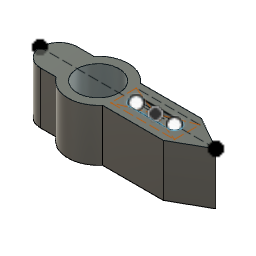
snafu-countdown-timer-arrow-v5 (Autodesk Fusion 360 design; units mm, degrees)
Autodesk Fusion 360 part; units mm, degrees
sketch "Sketch1" plane through (0, 0, 0) normal (0, 1, 0) x (1, 0, 0)
  line L0 (-20.3838, 3.2056) -> (-17.6853, 3.2056)
  line L1 (-20.3584, -2.5911) -> (-17.8516, -2.5911)
  line L2 (-10.3249, 3.1994) -> (-0.7249, 3.1994)
  line L3 (-0.7249, 3.1994) -> (4.589, 0.1994)
  line L4 (4.589, 0.1994) -> (-0.7249, -2.8006)
  line L5 (-0.7249, -2.8006) -> (-10.3249, -2.8006)
  arc A0 (-20.1646, 3.2056) -> (-20.19, -2.5911) centre (-20.2742, 0.3077) ccw
  arc A1 (-10.3249, 3.1994) -> (-17.6853, 3.2056) centre (-14.0077, 0.1994) ccw
  arc A2 (-17.8516, -2.5911) -> (-10.3249, -2.8006) centre (-14.0077, 0.1994) ccw
  line L6 (-22.911, 1.5149) -> (3.7873, -2.43) construction
  dimension "d1" = 5.8
  dimension "d2" = 9.5
  dimension "d4" = 27.5
  dimension "d32" = 6
  dimension "d33" = 9.6
  dimension "d34" = 9
  constraint coincident L0.start A0
  constraint horizontal L0
  constraint coincident L1.start A0
  constraint coincident L1.end A1
  constraint parallel L0 L1
  constraint coincident L6.start A0
  constraint parallel L0 L2
  constraint parallel L2 L5
  constraint concentric A1 A2
  constraint coincident L0 A0.start
  constraint coincident L1 A0.end
  constraint equal L3 L4
  constraint equal L2 L5
  constraint vertical L5.end L2.start
  constraint coincident A1.centre L6
  measures "d1" diameter of A0
  measures "d2" diameter of A1
  measures "d4" horizontal distance of L6.start L3.end
  measures "d32" distance of L2 L5
  measures "d33" distance of L2.end L2.start
  measures "d34" distance of A1.centre L6.start
extrude "Extrude1" add sketch "Sketch1" along normal blind 8.2
sketch "Sketch2" plane through (0, 8.2, 0) normal (0, 1, 0) x (-1, 0, 0)
  arc A0 (20.3838, -3.2056) -> (20.3584, 2.5911) centre (20.2742, -0.3077) ccw
  line L0 (20.3584, 2.5911) -> (17.8516, 2.5911)
  arc A1 (17.8516, 2.5911) -> (10.3249, 2.8006) centre (14.0077, -0.1994) ccw
  line L1 (10.3249, 2.8006) -> (0.7249, 2.8006)
  line L2 (0.7249, 2.8006) -> (-4.589, -0.1994)
  line L3 (-4.589, -0.1994) -> (0.7249, -3.1994)
  line L4 (0.7249, -3.1994) -> (10.3249, -3.1994)
  arc A2 (10.3249, -3.1994) -> (17.6853, -3.2056) centre (14.0077, -0.1994) ccw
  line L5 (17.6853, -3.2056) -> (20.3838, -3.2056)
  circle A3 centre (14.0077, -0.1994) radius 3.3
  dimension "d9" = 6.6
  constraint concentric A1 A3
  measures "d9" diameter of A3
extrude "Extrude2" cut sketch "Sketch2" against normal blind 5 contours A3
sketch "Sketch3" plane through (0, 3.2, 0) normal (0, 1, 0) x (-1, 0, 0)
  circle A0 centre (14.0077, -0.1994) radius 3.3
  line L0 (12.7077, -1.4994) -> (15.3077, -1.4994)
  line L1 (15.3077, -1.4994) -> (15.3077, 1.1006)
  line L2 (15.3077, 1.1006) -> (12.7077, 1.1006)
  line L3 (12.7077, 1.1006) -> (12.7077, -1.4994)
  line L4 (12.7077, -1.4994) -> (15.3077, 1.1006) construction
  line L5 (15.3077, -1.4994) -> (12.7077, 1.1006) construction
  point P0 (14.0077, -0.1994)
  dimension "d12" = 2.6
  constraint horizontal L0
  constraint perpendicular L0 L1
  constraint parallel L0 L2
  constraint parallel L1 L3
  constraint coincident L4 P0
  constraint coincident L5 P0
  constraint coincident P0 A0.centre
  constraint equal L1 L2
  measures "d12" distance of L0.end L1.end
extrude "Extrude3" cut sketch "Sketch3" against normal blind 13 contours L0 L1 L2 L3
sketch "Sketch6" plane through (0, 8.2, 0) normal (0, 1, 0) x (-1, 0, 0)
  circle A0 centre (14.0077, -0.1994) radius 3.3
  arc A1 (20.3838, -3.2056) -> (20.3584, 2.5911) centre (20.2742, -0.3077) ccw
  line L0 (20.3584, 2.5911) -> (17.8516, 2.5911)
  arc A2 (17.8516, 2.5911) -> (10.3249, 2.8006) centre (14.0077, -0.1994) ccw
  line L1 (10.3249, 2.8006) -> (0.7249, 2.8006)
  line L2 (0.7249, 2.8006) -> (-4.589, -0.1994)
  line L3 (-4.589, -0.1994) -> (0.7249, -3.1994)
  line L4 (0.7249, -3.1994) -> (10.3249, -3.1994)
  arc A3 (10.3249, -3.1994) -> (17.6853, -3.2056) centre (14.0077, -0.1994) ccw
  line L5 (17.6853, -3.2056) -> (20.3838, -3.2056)
  line L6 (-0.0396, -2.1994) -> (9.9928, -2.1994) construction
  line L7 (9.9928, -2.1994) -> (9.9928, 1.8006) construction
  line L8 (9.9928, 1.8006) -> (-0.0396, 1.8006) construction
  line L9 (-0.0396, 1.8006) -> (-0.0396, -2.1994) construction
  line L10 (-0.0396, -2.1994) -> (9.9928, 1.8006) construction
  line L11 (9.9928, -2.1994) -> (-0.0396, 1.8006) construction
  line L12 (7.9828, 0.8006) -> (1.9704, 0.8006)
  line L13 (0.9604, -0.2094) -> (0.9604, -0.1894)
  line L14 (1.9704, -1.1994) -> (7.9828, -1.1994)
  line L15 (8.9928, -0.1894) -> (8.9928, -0.2094)
  arc A4 (0.9604, -0.1894) -> (1.9704, -1.1994) centre (1.9704, -0.1894) ccw
  arc A5 (1.9704, 0.8006) -> (0.9604, -0.2094) centre (1.9704, -0.2094) ccw
  arc A6 (8.9928, -0.2094) -> (7.9828, 0.8006) centre (7.9828, -0.2094) ccw
  arc A7 (7.9828, -1.1994) -> (8.9928, -0.1894) centre (7.9828, -0.1894) ccw
  line L16 (-4.589, -0.1994) -> (8.9928, -0.1994) construction
  line L17 (9.9928, -0.1994) -> (23.1722, -0.1994) construction
  point P0 (4.9766, -0.1994)
  dimension "d28" = 1.01
  dimension "d29" = 2
  constraint coincident L2.end L3.start
  constraint coincident A1 L17.end
  constraint horizontal L16
  constraint horizontal L6
  constraint perpendicular L6 L7
  constraint parallel L6 L8
  constraint parallel L7 L9
  constraint coincident L10 P0
  constraint coincident L11 P0
  constraint coincident P0 L16
  constraint tangent L13 A4
  constraint tangent L14 A4
  constraint tangent L12 A5
  constraint tangent L13 A5
  constraint equal A4 A5
  constraint tangent L12 A6
  constraint tangent L15 A6
  constraint equal A4 A6
  constraint tangent L14 A7
  constraint tangent L15 A7
  constraint equal A4 A7
  constraint coincident L15 L16.end
  constraint coincident L7 L17.start
  constraint collinear L16 L17
  measures "d28" radius of A4
  measures "d29" distance of L4 L14
extrude "Extrude4" cut sketch "Sketch6" against normal blind 0.6 contours L12 L13 L14 L15 A4 A5 A6 A7
sketch "Sketch9" plane through (0, 0, 0) normal (0, -1, 0) x (1, 0, 0)
  line L0 (-12.7077, -1.4994) -> (-15.3077, -1.4994)
  line L1 (-15.3077, -1.4994) -> (-15.3077, 1.1006)
  line L2 (-15.3077, 1.1006) -> (-12.7077, 1.1006)
  line L3 (-12.7077, 1.1006) -> (-12.7077, -1.4994)
  arc A0 (-20.3584, 2.5911) -> (-20.3838, -3.2056) centre (-20.2742, -0.3077) ccw
  line L4 (-20.3838, -3.2056) -> (-17.6853, -3.2056)
  arc A1 (-17.6853, -3.2056) -> (-10.3249, -3.1994) centre (-14.0077, -0.1994) ccw
  line L5 (-10.3249, -3.1994) -> (-0.7249, -3.1994)
  line L6 (-0.7249, -3.1994) -> (4.589, -0.1994)
  line L7 (4.589, -0.1994) -> (-0.7249, 2.8006)
  line L8 (-0.7249, 2.8006) -> (-10.3249, 2.8006)
  arc A2 (-10.3249, 2.8006) -> (-17.8516, 2.5911) centre (-14.0077, -0.1994) ccw
  line L9 (-17.8516, 2.5911) -> (-20.3584, 2.5911)
  line L10 (-0.7249, -3.1994) -> (-10.3249, -3.1994)
  line L11 (-10.3249, 2.8006) -> (-0.7249, 2.8006)
  line L12 (-0.7249, 2.8006) -> (4.589, -0.1994)
  line L13 (4.589, -0.1994) -> (-0.7249, -3.1994)
  line L14 (-10.3249, -3.1994) -> (-10.3249, 2.8006) construction
  line L15 (-1.0403, -1.9994) -> (2.1481, -0.1994)
  line L16 (2.1481, -0.1994) -> (-1.0403, 1.6006)
  line L17 (-1.0403, 1.6006) -> (-9.1249, 1.6006)
  line L18 (-9.1249, -1.9994) -> (-9.1249, 1.6006)
  line L19 (-9.1249, -1.9994) -> (-1.0403, -1.9994)
  point P0 (-10.3249, -3.1994)
  point P1 (-0.7249, -3.1994)
  point P2 (4.589, -0.1994)
  point P3 (-0.7249, 2.8006)
  point P4 (-10.3249, 2.8006)
  dimension "d35" = -1.2
  constraint coincident P0 A1.end
  constraint coincident P4 L8.end
extrude "Extrude5" cut sketch "Sketch9" against normal blind 6 contours L15 L16 L17 L18 L19
fillet "Fillet1" radius 1.75 2 edges at (-9.1249, 3, 1.6006) (-9.1249, 3, -1.9994)
